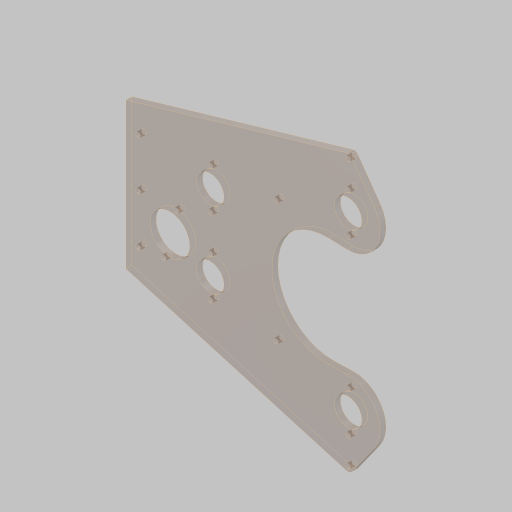
# Autodesk Inventor part: GP6-002
Saved by Autodesk Inventor 2023.5 (Build 275446000, 446)
## iProperties
Created: 2025-02-23
Part Number: GP6-002
Material: Polycarbonate, Smoke
Document SubType Name: Modeling
Designer: slick
Density: 1.2 g/cm^3
Appearance: Polycarbonate - Smoked
Author: slick
Autodesk Inventor part; units mm, degrees
ref_plane "YZ Plane" through (0, 0, 0) normal (1, 0, 0) x (0, 1, 0)
ref_plane "XZ Plane" through (0, 0, 0) normal (0, 1, 0) x (-1, 0, 0)
ref_plane "XY Plane" through (0, 0, 0) normal (0, 0, 1) x (1, 0, 0)
sketch "Sketch1" plane through (0, 0, 0) normal (0, 0, 1) x (1, 0, 0)
  circle A0 centre (0, 89.8026) radius 38.1 construction
  circle A1 centre (0, -89.8026) radius 38.1 construction
  line L0 (0, 89.8026) -> (0, -89.8026) construction
  circle A2 centre (-31.75, 0) radius 57.15 construction
  circle A3 centre (0, 89.8026) radius 14.2875
  circle A4 centre (0, -89.8026) radius 14.2875
  circle A5 centre (0, -89.8026) radius 33.3375 construction
  circle A6 centre (0, 89.8026) radius 33.3375 construction
  circle A7 centre (-143.7092, -39.6875) radius 14.3256 construction
  circle A8 centre (0, -89.8026) radius 23.876 construction
  line L1 (-143.7092, -39.6875) -> (0, -89.8026) construction
  circle A9 centre (-143.7092, 39.6875) radius 14.3256 construction
  circle A10 centre (0, 89.8026) radius 23.876 construction
  line L2 (0, 89.8026) -> (-143.7092, 39.6875) construction
  circle A11 centre (-143.7092, 39.6875) radius 39.6875 construction
  circle A12 centre (-143.7092, -39.6875) radius 39.6875 construction
  line L3 (-143.7092, 39.6875) -> (-143.7092, -39.6875) construction
  line L4 (-139.8502, 25.8915) -> (6.4317, 66.8092) construction
  line L5 (-9.261, 111.8093) -> (-149.2659, 52.8915) construction
  line L6 (-139.8502, -25.8915) -> (6.4317, -66.8092) construction
  line L7 (-13.2689, -109.652) -> (-135.7479, -27.7778) construction
  circle A13 centre (-143.7092, 39.6875) radius 14.2875
  circle A14 centre (-143.7092, -39.6875) radius 14.2875
  circle A15 centre (-185.8771, -22.225) radius 5.9531 construction
  circle A16 centre (-185.8771, -22.225) radius 9.525
  circle A17 centre (-185.8771, -22.225) radius 12.7 construction
  circle A18 centre (-185.8771, -22.225) radius 12.7 construction
  circle A19 centre (-185.8771, -22.225) radius 12.7 construction
  circle A20 centre (-185.8771, -22.225) radius 12.7 construction
  circle A21 centre (-185.8771, -22.225) radius 12.7 construction
  circle A22 centre (-22.225, 0) radius 57.15 construction
  circle A23 centre (-185.8771, -22.225) radius 20.6375
  line L8 (-231.775, 76.2) -> (-206.375, 76.2) construction
  line L9 (-206.375, 76.2) -> (-206.375, -76.2) construction
  line L10 (-206.375, -76.2) -> (-231.775, -76.2) construction
  line L11 (-231.775, -76.2) -> (-231.775, 76.2)
  line L12 (-143.7092, -39.6875) -> (-185.8771, -22.225) construction
  line L13 (-75.4249, 63.5) -> (-75.4249, -63.5) construction
  line L14 (-20.3378, -57.1188) -> (-1.1009, -56.4832)
  arc A24 (-1.1009, 56.4832) -> (27.142, 109.1598) centre (0, 89.8026) ccw
  arc A25 (-20.3378, 57.1188) -> (-20.3378, -57.1188) centre (-22.225, 0) ccw
  line L15 (-1.1009, 56.4832) -> (-20.3378, 57.1188)
  arc A26 (27.142, -109.1598) -> (-1.1009, -56.4832) centre (0, -89.8026) ccw
  arc A27 (3.8774, 141.7804) -> (-1.3367, 143.5861) centre (0, 139.0151) ccw
  circle A28 centre (0, 89.8026) radius 44.45 construction
  line L16 (3.8774, 141.7804) -> (27.142, 109.1598)
  line L17 (-1.3367, 143.5861) -> (-231.775, 76.2)
  arc A29 (-1.3367, -143.5861) -> (3.8774, -141.7804) centre (0, -139.0151) ccw
  line L18 (-231.775, -76.2) -> (-1.3367, -143.5861)
  line L19 (27.142, -109.1598) -> (3.8774, -141.7804)
  circle A30 centre (0, -89.8026) radius 44.45 construction
  line L20 (0, 110.8211) -> (0, 68.7841) construction
  line L21 (-143.7092, 60.706) -> (-143.7092, 18.669) construction
  line L22 (-143.7092, -18.669) -> (-143.7092, -60.706) construction
  line L23 (0, -68.7841) -> (0, -110.8211) construction
  line L24 (-219.075, 50.8) -> (-219.075, -50.8) construction
  line L25 (-179.3031, 2.3095) -> (-192.4511, -46.7595) construction
  point P0 (0, 0)
  point P1 (0, 0)
  point P2 (-173.1775, -22.1229)
  point P3 (-182.0498, -10.1154)
  point P4 (-196.2113, -14.843)
  point P5 (-196.0912, -29.7723)
  point P6 (-181.8556, -34.2715)
  point P7 (-206.375, 0)
  point P8 (-219.075, 0)
  point P9 (-219.075, 0)
  point P10 (-219.075, 76.2)
  dimension "d15" = 25.4
  dimension "d0" = 76.2
  dimension "d1" = 76.2
  dimension "d2" = 114.3
  dimension "d4" = 179.6051
  dimension "d5" = 28.575
  dimension "d6" = 19.05
  dimension "d7" = 28.6512
  dimension "d8" = 47.752
  dimension "d9" = 79.375
  dimension "d10" = 143.7092
  dimension "d11" = 152.1968
  dimension "d12" = 28.575
  dimension "d13" = 11.9062
  dimension "d14" = 19.05
  dimension "d18" = 360
  dimension "d20" = 9.525
  dimension "d21" = 41.275
  dimension "d22" = 25.4
  dimension "d23" = 152.4
  dimension "d24" = 231.775
  dimension "d26" = 127
  dimension "d29" = 9.525
  dimension "d30" = 6.35
  dimension "d32" = 42.037
  dimension "d33" = 42.037
  dimension "d34" = 42.037
  dimension "d35" = 42.037
  dimension "d36" = 31.75
  dimension "d44" = 101.6
  dimension "d45" = 53.975
  dimension "d46" = 50.8
  dimension "d47" = 15
  constraints: 52 end point, 26 centre point, 24 point on circle, 24 tangent, 19 coincident, 9 equal radius, 9 midpoint, 8 vertical, 3 horizontal alignment, 3 vertical alignment, 2 parallel, 2 point on line, 1 equal length, 1 horizontal, 1 perpendicular, 31 other
  measures "d0" diameter of A0
  measures "d1" diameter of A1
  measures "d2" diameter of A2
  measures "d4" distance of L0.start L0.end
  measures "d5" diameter of A3
  measures "d6" radial gap between concentric circles of A4 A5
  measures "d7" diameter of A7
  measures "d8" diameter of A8
  measures "d9" diameter of A11
  measures "d10" distance from line of L0.start L3
  measures "d11" distance of L2.end L2.start
  measures "d12" diameter of A13
  measures "d13" diameter of A15
  measures "d14" diameter of A16
  measures "d20" distance of A2.centre A22.centre
  measures "d21" diameter of A23
  measures "d22" distance of L9.end L10.end
  measures "d23" distance of L10.end L8.start
  measures "d24" distance from line of A3.centre L11
  measures "d26" distance of L13.start L13.end
  measures "d29" diameter of A27
  measures "d30" radial gap between concentric circles of A0 A28
  measures "d32" distance of L20.start L20.end
  measures "d33" distance of L21.start L21.end
  measures "d34" distance of L22.start L22.end
  measures "d35" distance of L23.start L23.end
  measures "d36" distance of point (0, 0) A2.centre
  measures "d44" distance of L24.start L24.end
  measures "d45" distance from line of L12.end L10
  measures "d46" distance of L25.start L25.end
  measures "d47" angle of L9 L25
extrude "Extrusion1" add sketch "Sketch1" along normal blind 6.35 contours L11 L17 A27 L16 A24 L15 A25 L14 A26 L19 A29 L18
hole "Hole1" at (-173.1775, -22.1229, 0) at (-182.0498, -10.1154, 0) at (-196.2113, -14.843, 0) at (-196.0912, -29.7723, 0) at (-181.8556, -34.2715, 0) at (-75.4249, 63.5, 0) at (-75.4249, -63.5, 0) at (0, 110.8211, 0) at (0, 68.7841, 0) at (-143.7092, 60.706, 0) at (-143.7092, 18.669, 0) at (-143.7092, -18.669, 0) at (-143.7092, -60.706, 0) at (0, -68.7841, 0) at (0, -110.8211, 0) at (-219.075, 50.8, 0) at (-219.075, 0, 0) at (-219.075, -50.8, 0) at (-192.4511, -46.7595, 0) at (-179.3031, 2.3095, 0) at (0, -139.0151, 0) at (0, 139.0151, 0) direction (0, 0, 1) diameter 5.1054 end through all clearance for "Flat Head Machine Screw (82)" size "#10" standard "Ansi Unified Screw Threads"
body "Solid1"
